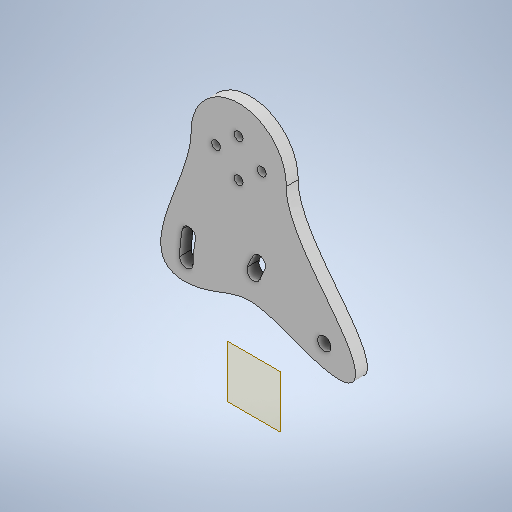
# Autodesk Inventor part: Soporte motor
Saved by Autodesk Inventor 2025.3 (Build 293356000, 356)
## iProperties
Created: 2025-11-12
Part Number: Soporte motor
Material: Generic
Document SubType Name: Modeling
Designer: juanm
Density: 1 g/cm^3
Appearance: Default
Author: juanm
Autodesk Inventor part; units mm, degrees
ref_plane "YZ Plane" through (0, 0, 0) normal (1, 0, 0) x (0, 1, 0)
ref_plane "XZ Plane" through (0, 0, 0) normal (0, 1, 0) x (-1, 0, 0)
ref_plane "XY Plane" through (0, 0, 0) normal (0, 0, 1) x (1, 0, 0)
sketch "Sketch1" plane through (0, 0, 0) normal (0, 0, 1) x (1, 0, 0)
  circle A0 centre (-25.0838, -31.7051) radius 2.5 projected
  circle A1 centre (-43.012, -13.2629) radius 2.5 projected
  circle A2 centre (-44.8914, 13.7567) radius 2.5 projected
  circle A3 centre (-28.0838, 36.7109) radius 2.5 construction
  circle A4 centre (0.8935, 43.7288) radius 2.5 construction
  circle A5 centre (29.5533, 30.4373) radius 2.5 projected
  circle A6 centre (43.6662, -0.0951) radius 2.5 projected
  circle A7 centre (47.6662, -52.5951) radius 2.5 projected
  circle A8 centre (10.6662, -52.5951) radius 2.5 projected
  circle A9 centre (-6.8338, -0.0951) radius 8.75 projected
  line L0 (56.6662, -60.0951) -> (51.1662, -0.0951) projected
  spline S0 degree 4 poles (51.1662, -0.0951) (50.0319, 24.6801) (26.25, 55.8136) (-25.1104, 60.0951) (-56.6662, 18.5311) (-54.7055, -22.2338) (-29.645, -43.1708) (-8.3823, -44.3792) (3.1662, -40.8213) knots 0 0 0 0 0 0.330099 0.457579 0.582312 0.704438 0.895347 0.895347 0.895347 0.895347 0.895347 projected
  line L1 (3.1662, -40.8213) -> (3.1662, -60.0951) projected
  line L2 (3.1662, -60.0951) -> (56.6662, -60.0951) projected
  circle A10 centre (-6.8338, -0.0951) radius 80 construction
  circle A11 centre (-6.409, 79.9037) radius 20
  spline S1 degree 4 poles (13.5883, 79.5717) (13.2828, 61.1776) (53.4159, 30.7093) (46.2466, 8.4135) (-3.1072, 37.0942) (-15.1022, 21.9833) (-58.6807, 16.6925) (-26.133, 63.1171) (-26.4062, 79.5717) knots 0 0 0 0 0 0.268909 0.429337 0.564159 0.731942 1 1 1 1 1
  arc A12 (2.161, 46.1761) -> (-0.1558, 41.1804) centre (29.5533, 30.4373) ccw
  arc A13 (-27.3177, 41.7105) -> (-28.4113, 31.6637) centre (29.5533, 30.4373) ccw
  line L3 (29.5533, 30.4373) -> (-27.3177, 41.7105) construction
  line L4 (-28.0838, 36.7109) -> (29.5533, 30.4373) construction
  line L5 (2.161, 46.1761) -> (29.5533, 30.4373) construction
  line L6 (-0.1558, 41.1804) -> (29.5533, 30.4373) construction
  line L7 (0.8935, 43.7288) -> (29.5533, 30.4373) construction
  line L8 (-28.4113, 31.6637) -> (29.5533, 30.4373) construction
  arc A14 (-30.9107, 31.7166) -> (-25.9118, 31.6108) centre (-28.4113, 31.6637) ccw
  arc A15 (-24.8654, 41.2244) -> (-29.77, 42.1966) centre (-27.3177, 41.7105) ccw
  arc A16 (4.3287, 44.9306) -> (-0.0066, 47.4216) centre (2.161, 46.1761) ccw
  arc A17 (-2.5068, 42.0305) -> (2.1952, 40.3302) centre (-0.1558, 41.1804) ccw
  arc A18 (-0.0066, 47.4216) -> (-2.5068, 42.0305) centre (29.5533, 30.4373) ccw
  arc A19 (4.3287, 44.9306) -> (2.1952, 40.3302) centre (29.5533, 30.4373) ccw
  arc A20 (-29.77, 42.1966) -> (-30.9118, 31.6637) centre (29.5533, 30.4373) ccw
  arc A21 (-24.8654, 41.2244) -> (-25.9118, 31.6108) centre (29.5533, 30.4373) ccw
  point P0 (0, 0)
  point P1 (42.6911, 26.1251)
  point P2 (35.4649, 20.4441)
  point P3 (1.223, 30.0999)
  point P4 (-17.2039, 26.1779)
  point P5 (-36.803, 26.1853)
  dimension "d0" = 160
  dimension "d1" = 40
  dimension "d4" = 5
  dimension "d5" = 5
  dimension "d6" = 5
  dimension "d7" = 5
  dimension "d8" = 5
  dimension "d9" = 5
  dimension "d10" = 5
  dimension "d11" = 5
  constraints: 25 point on circle, 12 end point, 11 centre point, 11 coincident, 4 tangent, 1 point on line, 12 other
  measures "d1" diameter of A11
  measures "d4" angle of L7 L5
  measures "d5" angle of L6 L7
  measures "d6" angle of L4 L3
  measures "d7" angle of L8 L4
  measures "d8" diameter of A14
  measures "d9" diameter of A15
  measures "d10" diameter of A17
  measures "d11" diameter of A16
ref_plane "Work Plane1" through (0, 0, 5) normal (0, 0, 1) x (1, 0, 0)
extrude "Extrusion2" add sketch "Sketch1" along normal blind 5 contours S1 S0 | S0 S1 A11 | A11
sketch "Sketch3" plane through (0, 0, 0) normal (0, 0, -1) x (-1, 0, 0)
  circle A0 centre (6.409, 79.9037) radius 20 projected
  circle A1 centre (6.409, 79.9037) radius 8 construction
  circle A2 centre (6.409, 79.9037) radius 9.5 construction
  point P0 (0, 0)
  point P1 (15.909, 79.9037)
  point P2 (6.409, 71.9037)
  point P3 (-3.3325, 79.9037)
  point P4 (6.409, 87.9037)
  dimension "d16" = 19
  dimension "d15" = 16
  constraints: 2 coincident, 2 point on circle, 1 centre point, 1 horizontal alignment, 2 other
  measures "d15" diameter of A1
hole "Hole1" at (-15.909, 79.9037, 0) at (-6.409, 71.9037, 0) at (3.3325, 79.9037, 0) at (-6.409, 87.9037, 0) direction (0, 0, 1) diameter 3.7 end through all
sketch "Sketch4" plane through (0, 0, 5) normal (0, 0, 1) x (1, 0, 0)
  circle A0 centre (3.3325, 79.9037) radius 1.85 projected
  circle A1 centre (-6.409, 71.9037) radius 1.85 projected
  circle A2 centre (-15.909, 79.9037) radius 1.85 projected
  circle A3 centre (-6.409, 87.9037) radius 1.85 projected
  circle A4 centre (3.3325, 79.9037) radius 4.5
  circle A5 centre (-6.409, 71.9037) radius 4.5
  circle A6 centre (-15.909, 79.9037) radius 4.5
  circle A7 centre (-6.409, 87.9037) radius 4.5
  point P0 (0, 0)
  dimension "d24" = 9
  dimension "d25" = 9
  dimension "d26" = 9
  dimension "d27" = 9
  constraints: 4 centre point, 4 coincident
  measures "d24" diameter of A4
  measures "d25" diameter of A5
  measures "d26" diameter of A6
  measures "d27" diameter of A7
extrude "Extrusion3" add sketch "Sketch4" against normal blind 7
sketch "Sketch5" plane through (0, 0, 0) normal (0, 0, -1) x (-1, 0, 0)
  circle A0 centre (-3.3325, 79.9037) radius 4.5 projected
  circle A1 centre (6.409, 71.9037) radius 4.5 projected
  circle A2 centre (6.409, 87.9037) radius 4.5 projected
  circle A3 centre (15.909, 79.9037) radius 4.5 projected
  arc A4 (26.4062, 79.5717) -> (-13.5883, 79.5717) centre (6.409, 79.9037) ccw projected
  arc A5 (25.9118, 31.6108) -> (24.8654, 41.2244) centre (-29.5533, 30.4373) ccw projected
  arc A6 (29.77, 42.1966) -> (24.8654, 41.2244) centre (27.3177, 41.7105) ccw projected
  arc A7 (30.9107, 31.7166) -> (29.77, 42.1966) centre (-29.5533, 30.4373) ccw projected
  arc A8 (25.9118, 31.6108) -> (30.9107, 31.7166) centre (28.4113, 31.6637) ccw projected
  circle A9 centre (-29.5533, 30.4373) radius 2.5 projected
  arc A10 (-2.1952, 40.3302) -> (-4.3287, 44.9306) centre (-29.5533, 30.4373) ccw projected
  arc A11 (0.0066, 47.4216) -> (-4.3287, 44.9306) centre (-2.161, 46.1761) ccw projected
  arc A12 (2.5068, 42.0305) -> (0.0066, 47.4216) centre (-29.5533, 30.4373) ccw projected
  arc A13 (-2.1952, 40.3302) -> (2.5068, 42.0305) centre (0.1558, 41.1804) ccw projected
  circle A14 centre (-29.5533, 30.4373) radius 2.8
  arc A15 (-2.4773, 40.2282) -> (-4.5888, 44.7812) centre (-29.5533, 30.4373) ccw
  arc A16 (-2.4773, 40.2282) -> (2.789, 42.1325) centre (0.1558, 41.1804) ccw
  arc A17 (2.789, 42.1325) -> (0.2668, 47.571) centre (-29.5533, 30.4373) ccw
  arc A18 (0.2668, 47.571) -> (-4.5888, 44.7812) centre (-2.161, 46.1761) ccw
  arc A19 (25.6119, 31.6044) -> (24.5711, 41.166) centre (-29.5533, 30.4373) ccw
  arc A20 (25.6119, 31.6044) -> (31.2106, 31.7229) centre (28.4113, 31.6637) ccw
  arc A21 (31.2106, 31.7229) -> (30.0643, 42.2549) centre (-29.5533, 30.4373) ccw
  arc A22 (30.0643, 42.2549) -> (24.5711, 41.166) centre (27.3177, 41.7105) ccw
  point P0 (0, 0)
  dimension "d30" = 0.3
  dimension "d31" = 0.3
  dimension "d32" = 0.3
  constraints: 16 point on circle, 9 centre point, 7 other
  measures "d30" radial gap between concentric circles of A9 A14
  measures "d31" radial gap between concentric circles of A10 A15
  measures "d32" radial gap between concentric circles of A5 A19
extrude "Extrusion4" cut sketch "Sketch5" against normal blind 7 contours A14 | A15 A18 A17 A16 | A19 A22 A21 A20
body "Solid2"
